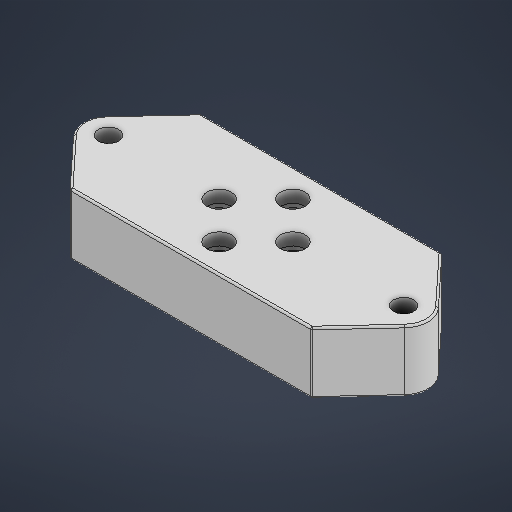
# Autodesk Inventor part: neck_v2
Saved by Autodesk Inventor 2026 (Build 300175000, 175)
## iProperties
Created: 2025-04-16
Part Number: neck_v2
Material: Generic
Document SubType Name: Modeling
Designer: Elizabeth
Density: 1 g/cm^3
Appearance: Default
Author: Elizabeth
Autodesk Inventor part; units mm, degrees
ref_plane "YZ Plane" through (0, 0, 0) normal (1, 0, 0) x (0, 1, 0)
ref_plane "XZ Plane" through (0, 0, 0) normal (0, 1, 0) x (-1, 0, 0)
ref_plane "XY Plane" through (0, 0, 0) normal (0, 0, 1) x (1, 0, 0)
sketch "Sketch1" plane through (0, 0, 0) normal (0, 1, 0) x (-1, 0, 0)
  circle A0 centre (-9, 0) radius 8.5
  circle A1 centre (15, 0) radius 4
  line L0 (10.6066, -10.6066) -> (17.9306, -2.7224)
  line L1 (10.6066, 10.6066) -> (17.9306, 2.7224)
  line L2 (16.6, -2.7713) -> (13.4, -2.7713)
  line L3 (13.4, -2.7713) -> (11.8, 0)
  line L4 (11.8, 0) -> (13.4, 2.7713)
  line L5 (13.4, 2.7713) -> (16.6, 2.7713)
  line L6 (16.6, 2.7713) -> (18.2, 0)
  line L7 (18.2, 0) -> (16.6, -2.7713)
  line L8 (15, -2.7713) -> (15, 2.7713)
  line L9 (11.8, 0) -> (15, 0)
  circle A2 centre (-9, 0) radius 6
  circle A3 centre (-9, -6) radius 1.2
  circle A4 centre (-15, 0) radius 1.2
  circle A5 centre (-9, 6) radius 1.2
  circle A6 centre (-3, 0) radius 1.2
  circle A7 centre (15, 0) radius 1.65
  line L10 (11, 0) -> (-29, 0)
  circle A8 centre (-33, 0) radius 4
  line L11 (-28.6066, -10.6066) -> (-35.9306, -2.7224)
  line L12 (-28.6066, 10.6066) -> (-35.9306, 2.7224)
  line L13 (-31.4, -2.7713) -> (-34.6, -2.7713)
  line L14 (-34.6, -2.7713) -> (-36.2, 0)
  line L15 (-36.2, 0) -> (-34.6, 2.7713)
  line L16 (-36.2, 0) -> (-33, 0)
  line L17 (-33, -2.7713) -> (-33, 2.7713)
  line L18 (-34.6, 2.7713) -> (-31.4, 2.7713)
  line L19 (-29.8, 0) -> (-31.4, -2.7713)
  line L20 (-31.4, 2.7713) -> (-29.8, 0)
  circle A9 centre (-33, 0) radius 1.65
  line L21 (-28.6066, -10.6066) -> (10.6066, -10.6066)
  line L22 (-28.6066, 10.6066) -> (10.6066, 10.6066)
  dimension "d49" = 4
  dimension "d55" = 8
  dimension "d22" = 3.2
  dimension "d34" = 12
  dimension "d35" = 2.4
  dimension "d36" = 2.4
  dimension "d37" = 2.4
  dimension "d38" = 2.4
  dimension "d43" = 3.3
  dimension "d54" = 40
  dimension "d56" = 3.2
  dimension "d57" = 3.2
  dimension "d58" = 120
  dimension "d59" = 3.2
  dimension "d60" = 120
  dimension "d61" = 3.3
  constraints: 46 end point, 9 centre point, 6 horizontal, 6 midpoint, 6 point on circle, 3 coincident, 1 parallel, 1 tangent, 3 other
  measures "d22" distance of L2.start L2.end
  measures "d34" diameter of A2
  measures "d35" diameter of A3
  measures "d36" diameter of A4
  measures "d37" diameter of A5
  measures "d38" diameter of A6
  measures "d43" diameter of A7
  measures "d54" distance of L10.start L10.end
  measures "d56" distance of L19.end L14.start
  measures "d57" distance of L14.start L15.start
  measures "d58" angle of L13 L14
  measures "d59" distance of L15.start L15.end
  measures "d60" angle of L14 L15
  measures "d61" diameter of A9
extrude "Extrusion1" add sketch "Sketch1" along normal blind 10 contours L10 A6 A2 A5 A4 A0 | L10 A1 L0 L21 L11 A8 A0 | A0 L10 A8 L12 L22 L1 A1 | A0 L10 A4 A2 A3 A6 | A1 | L10 A2 A6 | A6 A2 L10 | L10 A2 A4 | A4 A2 L10 | A8 | A6 L10 A4 A2 A5 | A2 L10 A6 | A6 L10 A2 | A2 A3 A4 L10 A6 | A4 L10 A2 | A2 L10 A4 | A5 A2 | A2 A5 | A3 A2 | A2 A3 | L2 L8 A7 L5 L6 L7 | L2 L3 L9 A7 L8 | A7 L9 L8 | L8 A7 | L4 L5 L8 A7 L9 | L9 A7 L8 | L13 L17 A9 L18 L20 L19 | L13 L14 L16 A9 L17 | A9 L16 L17 | L17 A9 | L15 L18 L17 A9 L16 | L16 A9 L17
extrude "Extrusion2" cut sketch "Sketch1" along normal blind 2.5 contours L10 A6 A2 A5 A4 A0 | A0 L10 A4 A2 A3 A6 | L10 A2 A6 | A6 A2 L10 | L10 A2 A4 | A4 A2 L10 | A6 L10 A4 A2 A5 | A2 L10 A6 | A6 L10 A2 | A2 A3 A4 L10 A6 | A4 L10 A2 | A2 L10 A4 | A5 A2 | A2 A5 | A3 A2 | A2 A3 | L2 L8 A7 L5 L6 L7 | L2 L3 L9 A7 L8 | A7 L9 L8 | L8 A7 | L4 L5 L8 A7 L9 | L9 A7 L8 | L13 L17 A9 L18 L20 L19 | L13 L14 L16 A9 L17 | A9 L16 L17 | L17 A9 | L15 L18 L17 A9 L16 | L16 A9 L17
extrude "Extrusion3" cut sketch "Sketch1" along normal blind 10 contours L10 A2 A6 | A6 A2 L10 | L10 A2 A4 | A4 A2 L10 | A2 L10 A6 | A6 L10 A2 | A4 L10 A2 | A2 L10 A4 | A5 A2 | A2 A5 | A3 A2 | A2 A3 | A7 L9 L8 | L8 A7 | L9 A7 L8 | A9 L16 L17 | L17 A9 | L16 A9 L17
fillet "Fillet1" radius 0.3 20 edges at (-19, 0, 0) (-14.2686, 0, 6.6645) (-14.2686, 0, -6.6645) (-19, 10, 0) (-14.2686, 10, 6.6645) (-14.2686, 10, -6.6645) (9, 10, 10.6066) (9, 0, 10.6066) (9, 10, -10.6066) (9, 0, -10.6066) (-10.6066, 5, -10.6066) (-10.6066, 5, 10.6066) (37, 0, 0) (32.2686, 0, -6.6645) (32.2686, 0, 6.6645) (37, 10, 0) (32.2686, 10, -6.6645) (32.2686, 10, 6.6645) (28.6066, 5, -10.6066) (28.6066, 5, 10.6066)
sketch "Sketch2" plane through (0, 10, 0) normal (0, 1, 0) x (1, 0, 0)
  circle A0 centre (3, 0) radius 1.2 projected
  circle A1 centre (3, 0) radius 2
  circle A2 centre (9, 6) radius 1.2 projected
  circle A3 centre (9, 6) radius 2
  circle A4 centre (15, 0) radius 1.2 projected
  circle A5 centre (15, 0) radius 2
  circle A6 centre (9, -6) radius 1.2 projected
  circle A7 centre (9, -6) radius 2
  point P0 (0, 0)
  dimension "d22" = 3.2
  dimension "d43" = 3.3
  dimension "d48" = 4
  dimension "d49" = 4
  dimension "d50" = 4
  dimension "d51" = 4
  constraints: 4 centre point, 4 coincident
  measures "d48" diameter of A1
  measures "d49" diameter of A3
  measures "d50" diameter of A5
  measures "d51" diameter of A7
extrude "Extrusion5" cut sketch "Sketch2" against normal blind 2 contours A0 | A1 | A2 | A3 | A4 | A5 | A6 | A7
body "Solid1"
